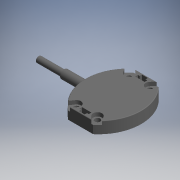
# Autodesk Inventor part: Abdeckkappe_LZ80_funkprofil
Saved by Autodesk Inventor 2021 (Build 250183000, 183)
## iProperties
Part Number: Abdeckkappe_LZ80_funkprofil
Material: Generic
Catalog Web Link: www.cadenas.de
Description: LZ80 Abdeckkappe Funktionsprofil-Bauteil LZ80
Vendor: ROSEKRIEGER
Document SubType Name: Modeling
Designer: partserver
Manufacturer: ROSEKRIEGER
Mass: 186.395 g
Surface Area: 318.535 cm^2
Volume: 186.395 cm^3
Density: 1 g/cm^3
Appearance: PSOLRGB-128-128-128
Category: PARTsolutions
Company: ROSEKRIEGER
PSOL_IDENT_0: {$CADENAS_DATA\23d-libs\rose_krieger\linearkomponenten\pool_lineartechnik\_hubsaeule_zyliinder\elekt
PSOL_IDENT_1: rozylinder\elekzyl_lz80\lz80_abdeckkappe_funktionsprofil.prj},211 {VTYP=3D},{NB=Abdeckkappe_LZ80_fun
PSOL_IDENT_2: kprofil},{LINA=Abdeckkappe_LZ80_funkprofil},{NN=LZ80 Abdeckkappe Funktionsprofil},{DATE=02.12.2020 1
PSOL_IDENT_3: 1:16:40},{GEOMDATE=12.12.2006},{VERSION=},{LINEID=10},{WBVAR=},{WBNUMERIC=}  {NB=Abdeckkappe_LZ80_fu
PSOL_IDENT_4: nkprofil},{LINA=Abdeckkappe_LZ80_funkprofil},{KT=DUMMY},{IDNR=},{ARTIKEL=Abdeckkappe_LZ80_funkprofil
PSOL_IDENT_5: },{BREITE=112.000},{HOEKAP=20.000},{XRADKONTUR=25.250},{RADKONTUR=72.950},{GESHOE=26.500},{ZENTA=56.
PSOL_IDENT_6: 000},{ZENTB=50.500},{TIEFZENTB=6.000},{TIEFZENTA=5.500},{DURCHA=50.000},{ZENTC=44.000},{TIEFZENTC=20
PSOL_IDENT_7: .000},{RADIUS2=0.500},{RADIUS3=1.000},{DURCHB=41.500},{NUTBR1=16.000},{NUTBR2=10.000},{NUTTIEFE1=8.5
PSOL_IDENT_8: 00},{NUTTIEFE2=4.500},{NUTAB=2.000},{SENKDURCHB=9.000},{ABSENKLAE=90.000},{ABSENKBR=36.000},{SENKDUR
PSOL_IDENT_9: CHT=6.400},{SENKDURCHK=15.000},{WINKPUNKT=18.300},{WINKPUNKT2=29.300},{BRKABEL=17.000},{HOEKABEL=2.8
PSOL_IDENT_10: 00},{DLEITSCHUT=14.500},{DLEIT=10.000},{LLEITSCHU=33.500},{LLEIT=10.000}
NB: Abdeckkappe_LZ80_funkprofil
NN: LZ80 Abdeckkappe Funktionsprofil
NT: Bauteil LZ80
NBSYN: $ARTIKEL.
LINA: Abdeckkappe_LZ80_funkprofil
CATALOG: RK Rose+Krieger
ARTIKEL: Abdeckkappe_LZ80_funkprofil
BREITE: 112
HOEKAP: 20
XRADKONTUR: 25.25
RADKONTUR: 72.95
GESHOE: 26.5
ZENTA: 56
ZENTB: 50.5
TIEFZENTB: 6
TIEFZENTA: 5.5
DURCHA: 50
ZENTC: 44
TIEFZENTC: 20
RADIUS2: 0.5
RADIUS3: 1
DURCHB: 41.5
NUTBR1: 16
NUTBR2: 10
NUTTIEFE1: 8.5
NUTTIEFE2: 4.5
NUTAB: 2
SENKDURCHB: 9
ABSENKLAE: 90
ABSENKBR: 36
SENKDURCHT: 6.4
SENKDURCHK: 15
WINKPUNKT: 18.3
WINKPUNKT2: 29.3
BRKABEL: 17
HOEKABEL: 2.8
DLEITSCHUT: 14.5
DLEIT: 10
LLEITSCHU: 33.5
LLEIT: 10
SUPPLIER: ROSEKRIEGER
ARTICLENO: Abdeckkappe_LZ80_funkprofil
BOMINFO: Abdeckkappe_LZ80_funkprofil
CREATOR: CADENAS GmbH
Title: Abdeckkappe_LZ80_funkprofil
Author: Cadenas PARTsolutions
Comments: Bauteil LZ80
Autodesk Inventor part; units mm, degrees
sketch "Skizze_1" plane through (0, 0, 0) normal (0, 0, 1) x (1, 0, 0)
  arc A0 (-21.5015, 56) -> (-21.5015, -56) centre (25.25, 0) ccw
  line L0 (-21.5015, -56) -> (21.5015, -56)
  arc A1 (21.5015, -56) -> (21.5015, 56) centre (-25.25, 0) ccw
  line L1 (21.5015, 56) -> (-21.5015, 56)
  constraints: 4 end point, 4 point on circle, 2 centre point
extrude "Extrusion1" add sketch "Skizze_1" along normal blind 20
sketch "Skizze_2" plane through (0, 0, 0) normal (0, 1, 0) x (-1, 0, 0)
  line L0 (-25.25, -50) -> (-25.25, 50)
  line L1 (48.2, -0.5) -> (48.2, 1)
  line L2 (48.2, 1) -> (47.7, 1)
  arc A0 (46.7, 0) -> (47.7, 1) centre (46.7, 1) ccw
  line L3 (46.7, 0) -> (46.7, -0.5)
  line L4 (46.7, -0.5) -> (48.2, -0.5)
  constraints: 10 end point, 2 point on circle, 1 centre point
revolve "Revolution1" cut sketch "Skizze_2" angle 360 about axis through (25.25, 0, -50) along (0, 0, -1)
sketch "Skizze_3" plane through (0, 0, 0) normal (0, 1, 0) x (-1, 0, 0)
  line L0 (25.25, 50) -> (25.25, -50)
  arc A0 (-47.7, 1) -> (-46.7, 0) centre (-46.7, 1) ccw
  line L1 (-47.7, 1) -> (-48.2, 1)
  line L2 (-48.2, 1) -> (-48.2, -0.5)
  line L3 (-48.2, -0.5) -> (-46.7, -0.5)
  line L4 (-46.7, -0.5) -> (-46.7, 0)
  constraints: 10 end point, 2 point on circle, 1 centre point
revolve "Revolution2" cut sketch "Skizze_3" angle 360 about axis through (-25.25, 0, 50) along (0, 0, 1)
sketch "Skizze_4" plane through (0, 0, 0) normal (1, 0, 0) x (0, 1, 0)
  arc A0 (55, 0) -> (56, 1) centre (55, 1) ccw
  line L0 (55, 0) -> (56, 0)
  line L1 (56, 0) -> (56, 1)
  constraints: 4 end point, 2 point on circle, 1 centre point
extrude "Extrusion2" cut sketch "Skizze_4" along normal mid plane 112
sketch "Skizze_5" plane through (0, 0, 0) normal (1, 0, 0) x (0, 1, 0)
  line L0 (-56, 1) -> (-56, 0)
  line L1 (-56, 0) -> (-55, 0)
  arc A0 (-56, 1) -> (-55, 0) centre (-55, 1) ccw
  constraints: 4 end point, 2 point on circle, 1 centre point
extrude "Extrusion3" cut sketch "Skizze_5" along normal mid plane 112
sketch "Skizze_6" plane through (0, 0, 0) normal (0, 0, 1) x (1, 0, 0)
  circle A0 centre (0, 0) radius 25
  constraints: 1 centre point
extrude "Extrusion4" add sketch "Skizze_6" along normal blind 26.5
sketch "Skizze_8" plane through (0, 0, 0) normal (0, 0, 1) x (1, 0, 0)
  line L0 (-8, 50) -> (-8, 45.5)
  line L1 (-8, 45.5) -> (8, 45.5)
  line L2 (8, 45.5) -> (8, 50)
  line L3 (8, 50) -> (5, 50)
  line L4 (5, 50) -> (5, 54)
  line L5 (5, 54) -> (-5, 54)
  line L6 (-5, 54) -> (-5, 50)
  line L7 (-5, 50) -> (-8, 50)
  constraints: 16 end point
extrude "Extrusion5" cut sketch "Skizze_8" along normal blind 20
sketch "Skizze_9" plane through (0, 0, 0) normal (0, 0, 1) x (1, 0, 0)
  line L0 (-8, -45.5) -> (-8, -50)
  line L1 (-8, -50) -> (-5, -50)
  line L2 (-5, -50) -> (-5, -54)
  line L3 (-5, -54) -> (5, -54)
  line L4 (5, -54) -> (5, -50)
  line L5 (5, -50) -> (8, -50)
  line L6 (8, -50) -> (8, -45.5)
  line L7 (8, -45.5) -> (-8, -45.5)
  constraints: 16 end point
extrude "Extrusion6" cut sketch "Skizze_9" along normal blind 20
sketch "Skizze_10" plane through (0, 0, 6.4) normal (0, 0, 1) x (1, 0, 0)
  circle A0 centre (18, 45) radius 4.5
  constraints: 1 centre point
extrude "Extrusion7" cut sketch "Skizze_10" along normal mid plane 40
pattern_linear "Rectangular Pattern1" count 2 spacing 36 along (-1, 0, 0) count 2 spacing 90 along (0, -1, 0) of "Extrusion7"
sketch "Skizze_12" plane through (0, 0, 6.4) normal (0, 0, 1) x (1, 0, 0)
  arc A0 (12.6532, 50.2595) -> (24.242, 40.8422) centre (18, 45) ccw
  line L0 (24.242, 40.8422) -> (29.3, 48.4355)
  arc A1 (29.3, 48.4355) -> (21.5015, 56) centre (-25.25, 0) ccw
  line L1 (21.5015, 56) -> (18.3, 56)
  line L2 (18.3, 56) -> (12.6532, 50.2595)
  constraints: 6 end point, 4 point on circle, 2 centre point
extrude "Extrusion8" cut sketch "Skizze_12" against normal blind 6.4
sketch "Skizze_13" plane through (0, 0, 6.4) normal (0, 0, 1) x (1, 0, 0)
  line L0 (-29.3, 48.4355) -> (-24.242, 40.8422)
  arc A0 (-24.242, 40.8422) -> (-12.6532, 50.2595) centre (-18, 45) ccw
  line L1 (-12.6532, 50.2595) -> (-18.3, 56)
  line L2 (-18.3, 56) -> (-21.5015, 56)
  arc A1 (-21.5015, 56) -> (-29.3, 48.4355) centre (25.25, 0) ccw
  constraints: 6 end point, 4 point on circle, 2 centre point
extrude "Extrusion9" cut sketch "Skizze_13" against normal blind 6.4
sketch "Skizze_14" plane through (0, 0, 6.4) normal (0, 0, 1) x (1, 0, 0)
  arc A0 (24.242, -40.8422) -> (12.6532, -50.2595) centre (18, -45) ccw
  line L0 (12.6532, -50.2595) -> (18.3, -56)
  line L1 (18.3, -56) -> (21.5015, -56)
  arc A1 (21.5015, -56) -> (29.3, -48.4355) centre (-25.25, 0) ccw
  line L2 (29.3, -48.4355) -> (24.242, -40.8422)
  constraints: 6 end point, 4 point on circle, 2 centre point
extrude "Extrusion10" cut sketch "Skizze_14" against normal blind 6.4
sketch "Skizze_15" plane through (0, 0, 6.4) normal (0, 0, 1) x (1, 0, 0)
  arc A0 (-29.3, -48.4355) -> (-21.5015, -56) centre (25.25, 0) ccw
  line L0 (-21.5015, -56) -> (-18.3, -56)
  line L1 (-18.3, -56) -> (-12.6532, -50.2595)
  arc A1 (-12.6532, -50.2595) -> (-24.242, -40.8422) centre (-18, -45) ccw
  line L2 (-24.242, -40.8422) -> (-29.3, -48.4355)
  constraints: 6 end point, 4 point on circle, 2 centre point
extrude "Extrusion11" cut sketch "Skizze_15" against normal blind 6.4
sketch "Skizze_7" plane through (0, 0, 0) normal (1, 0, 0) x (0, 1, 0)
  line L0 (8.5, 20) -> (-8.5, 20)
  line L1 (-8.5, 20) -> (-8.5, 11.5)
  arc A0 (-8.5, 11.5) -> (8.5, 11.5) centre (0, 11.5) ccw
  line L2 (8.5, 11.5) -> (8.5, 20)
  constraints: 6 end point, 2 point on circle, 1 centre point
extrude "Extrusion12" add sketch "Skizze_7" along normal blind 50.5
sketch "Skizze_16" plane through (0, 0, 0) normal (0, 1, 0) x (-1, 0, 0)
  line L0 (-127.5, 11.5) -> (0, 11.5)
  line L1 (0, 11.5) -> (0, 4.25)
  line L2 (0, 4.25) -> (-84, 4.25)
  line L3 (-84, 4.25) -> (-84, 6.5)
  line L4 (-84, 6.5) -> (-127.5, 6.5)
  line L5 (-127.5, 6.5) -> (-127.5, 11.5)
  line L6 (-127.5, 11.5) -> (0, 11.5)
  constraints: 14 end point
revolve "Revolution3" add sketch "Skizze_16" angle 360 about axis through (127.5, 0, 11.5) along (1, 0, 0)
ref_plane "EPKAPPE_XY" through (0, 0, 20) normal (0, 0, 1) x (1, 0, 0)
ref_plane "EPKAPPE_YZ" through (0, 0, 20) normal (1, 0, 0) x (0, 1, 0)
ref_plane "EPKAPPE_ZX" through (0, 0, 20) normal (0, 1, 0) x (0, 0, 1)
ref_plane "EPZYL1_XY" through (18, 45, 6.4) normal (0, 0, 1) x (1, 0, 0)
ref_plane "EPZYL1_YZ" through (18, 45, 6.4) normal (1, 0, 0) x (0, 1, 0)
ref_plane "EPZYL1_ZX" through (18, 45, 6.4) normal (0, 1, 0) x (0, 0, 1)
ref_plane "EPZYL2_XY" through (-18, 45, 6.4) normal (0, 0, 1) x (1, 0, 0)
ref_plane "EPZYL2_YZ" through (-18, 45, 6.4) normal (1, 0, 0) x (0, 1, 0)
ref_plane "EPZYL2_ZX" through (-18, 45, 6.4) normal (0, 1, 0) x (0, 0, 1)
ref_plane "EPZYL3_XY" through (-18, -45, 6.4) normal (0, 0, 1) x (1, 0, 0)
ref_plane "EPZYL3_YZ" through (-18, -45, 6.4) normal (1, 0, 0) x (0, 1, 0)
ref_plane "EPZYL3_ZX" through (-18, -45, 6.4) normal (0, 1, 0) x (0, 0, 1)
ref_plane "EPZYL4_XY" through (18, -45, 6.4) normal (0, 0, 1) x (1, 0, 0)
ref_plane "EPZYL4_YZ" through (18, -45, 6.4) normal (1, 0, 0) x (0, 1, 0)
ref_plane "EPZYL4_ZX" through (18, -45, 6.4) normal (0, 1, 0) x (0, 0, 1)
body "Solid1"
